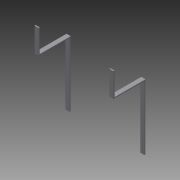
# Autodesk Inventor part: SideArm
Saved by Autodesk Inventor 2013 (Build 170138000, 138)
## iProperties
Created: 2014-01-09
Part Number: SideArm
Material: Generic
Document SubType Name: Modeling
Designer: 215152
Density: 1 g/cm^3
Author: 215152
Autodesk Inventor part; units mm, degrees
ref_plane "YZ Plane" through (0, 0, 0) normal (1, 0, 0) x (0, 1, 0)
ref_plane "XZ Plane" through (0, 0, 0) normal (0, 1, 0) x (-1, 0, 0)
ref_plane "XY Plane" through (0, 0, 0) normal (0, 0, 1) x (1, 0, 0)
sketch "Sketch1" plane through (0, 0, 0) normal (0, 0, 1) x (1, 0, 0)
  line L0 (0, 0) -> (76.2, 0)
  line L1 (76.2, 0) -> (76.2, 76.2)
  line L2 (76.2, 76.2) -> (0, 76.2)
  line L3 (0, 76.2) -> (0, 0)
  line L4 (76.2, 76.2) -> (167.64, 76.2)
  line L5 (167.64, 76.2) -> (594.36, 76.2)
  line L6 (594.36, 76.2) -> (685.8, 76.2)
  line L7 (167.64, 76.2) -> (594.36, 76.2)
  line L8 (594.36, 76.2) -> (594.36, -406.4)
  line L9 (594.36, -406.4) -> (167.64, -406.4)
  line L10 (167.64, -406.4) -> (167.64, 76.2)
  line L11 (167.64, -406.4) -> (142.24, -406.4)
  line L12 (142.24, -406.4) -> (142.24, 76.2)
  line L13 (142.24, 76.2) -> (167.64, 76.2)
  line L14 (167.64, 76.2) -> (167.64, -406.4)
  line L15 (594.36, 76.2) -> (619.76, 76.2)
  line L16 (619.76, 76.2) -> (619.76, -406.4)
  line L17 (619.76, -406.4) -> (594.36, -406.4)
  line L18 (594.36, -406.4) -> (594.36, 76.2)
  dimension "d0" = 76.2
  dimension "d1" = 76.2
  dimension "d2" = 91.44
  dimension "d3" = 426.72
  dimension "d4" = 91.44
  dimension "d5" = 426.72
  dimension "d6" = 482.6
  dimension "d7" = 25.4
  dimension "d8" = 482.6
  dimension "d9" = 25.4
  dimension "d10" = 482.6
  constraints: 38 end point, 8 parallel, 5 perpendicular, 4 horizontal, 2 collinear
  measures "d0" distance of L2.end L1.end
  measures "d1" distance of L1.end L0.end
  measures "d2" distance of L1.end L4.end
  measures "d3" distance of L4.end L5.end
  measures "d4" distance of L5.end L6.end
  measures "d5" distance of L8.end L9.end
  measures "d6" distance of L7.end L8.end
  measures "d7" distance of L12.end L13.end
  measures "d8" distance of L11.end L12.end
  measures "d9" distance of L16.end L17.end
  measures "d10" distance of L15.end L16.end
extrude "Extrusion1" add sketch "Sketch1" along normal blind 19.05 contours L4 L10 L11 L12 | L6 L16 L17 L8
sketch "Sketch2" plane through (142.24, -406.4, 0) normal (-1, 0, 0) x (0, 0, 1)
  line L0 (0, 482.6) -> (12.7, 482.6)
  line L1 (12.7, 482.6) -> (12.7, 0)
  line L2 (12.7, 0) -> (0, 0)
  line L3 (0, 0) -> (0, 482.6)
  point P0 (0, 406.4)
  dimension "d13" = 12.7
  dimension "d14" = 482.6
  constraints: 8 end point, 2 parallel, 1 horizontal, 1 perpendicular
  measures "d13" distance of L1.end L2.end
  measures "d14" distance of L0.end L1.end
extrude "Extrusion2" cut sketch "Sketch2" against normal blind 2090.7375
sketch "Sketch3" plane through (619.76, -406.4, 19.05) normal (1, 0, 0) x (0, 0, -1)
  line L0 (19.05, 406.4) -> (6.35, 406.4)
  line L1 (6.35, 406.4) -> (6.35, 393.7)
  line L2 (6.35, 393.7) -> (19.05, 393.7)
  line L3 (19.05, 393.7) -> (19.05, 406.4)
  line L4 (6.35, 393.7) -> (193.675, 393.7)
  line L5 (193.675, 393.7) -> (193.675, 387.35)
  line L6 (193.675, 387.35) -> (6.35, 387.35)
  line L7 (6.35, 387.35) -> (6.35, 393.7)
  line L8 (193.675, 387.35) -> (187.325, 387.35)
  line L9 (187.325, 387.35) -> (187.325, 0)
  line L10 (187.325, 0) -> (193.675, 0)
  line L11 (193.675, 0) -> (193.675, 387.35)
  dimension "d17" = 12.7
  dimension "d18" = 12.7
  dimension "d19" = 187.325
  dimension "d20" = 6.35
  dimension "d21" = 6.35
  dimension "d22" = 387.35
  constraints: 24 end point, 6 parallel, 3 horizontal, 3 perpendicular
  measures "d17" distance of L2.end L1.end
  measures "d18" distance of L1.end L0.end
  measures "d19" distance of L5.end L6.end
  measures "d20" distance of L4.end L5.end
  measures "d21" distance of L10.end L9.end
  measures "d22" distance of L9.end L8.end
extrude "Extrusion3" add sketch "Sketch3" against normal blind 477.52 contours L4 L5 L6 L7 L2 | L11 L10 L9 L6
sketch "Sketch4" plane through (142.24, -406.4, 19.05) normal (-1, 0, 0) x (0, 0, 1)
  line L0 (-6.35, 387.35) -> (0, 387.35)
  line L1 (0, 387.35) -> (0, 0)
  line L2 (0, 0) -> (-6.35, 0)
  line L3 (-6.35, 0) -> (-6.35, 387.35)
  point P0 (-19.05, 406.4)
  constraints: 8 end point, 2 parallel, 1 horizontal, 1 perpendicular
extrude "Extrusion4" cut sketch "Sketch4" against normal blind 684.53
sketch "Sketch5" plane through (167.64, -19.05, 12.7) normal (0, 0, 1) x (1, 0, 0)
  line L0 (0, 0) -> (0, 6.35) projected
  line L1 (426.72, 0) -> (0, 0) projected
  line L2 (426.72, 6.35) -> (426.72, 0) projected
  line L3 (426.72, 6.35) -> (0, 6.35) projected
  point P0 (-167.64, 19.05)
extrude "Extrusion5" cut sketch "Sketch5" against normal blind 1007.745
sketch "Sketch6" plane through (619.76, -406.4, -168.275) normal (0, 0, 1) x (1, 0, 0)
  line L0 (0, 0) -> (-477.52, 0) projected
  line L1 (-452.12, 387.35) -> (-25.4, 387.35)
  line L2 (-25.4, 387.35) -> (-25.4, 0)
  line L3 (-25.4, 0) -> (-452.12, 0)
  line L4 (-452.12, 0) -> (-452.12, 387.35)
  point P0 (-619.76, 406.4)
  constraints: 8 end point, 2 parallel, 1 horizontal, 1 perpendicular, 1 point on line
extrude "Extrusion6" cut sketch "Sketch6" against normal blind 187.6425
sketch "Sketch7" plane through (594.36, 76.2, 19.05) normal (0, 1, 0) x (1, 0, 0)
  line L0 (25.4, 6.35) -> (0, 6.35) projected
  line L1 (0, 6.35) -> (0, 0) projected
  line L2 (25.4, 0) -> (0, 0) projected
  line L3 (25.4, 6.35) -> (25.4, 0) projected
  point P0 (-594.36, 19.05)
extrude "Extrusion7" add sketch "Sketch7" along normal blind 50.8
sketch "Sketch8" plane through (142.24, 76.2, 19.05) normal (0, 1, 0) x (1, 0, 0)
  line L0 (25.4, 6.35) -> (0, 6.35) projected
  line L1 (0, 6.35) -> (0, 0) projected
  line L2 (25.4, 0) -> (0, 0) projected
  line L3 (25.4, 6.35) -> (25.4, 0) projected
  point P0 (-142.24, 19.05)
extrude "Extrusion8" add sketch "Sketch8" along normal blind 50.8
body "Solid1"
